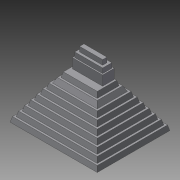
# Autodesk Inventor part: Basic Temple
Saved by Autodesk Inventor 2015 (Build 190159000, 159)
## iProperties
Created: 2016-11-16
Part Number: Basic Temple
Material: Generic
Document SubType Name: Modeling
Designer: Simms
Density: 1 g/cm^3
Appearance: Default
Author: Simms
Autodesk Inventor part; units mm, degrees
ref_plane "YZ Plane" through (0, 0, 0) normal (1, 0, 0) x (0, 1, 0)
ref_plane "XY Plane" through (0, 0, 0) normal (0, 0, 1) x (1, 0, 0)
sketch "Sketch1" plane through (0, 0, 0) normal (0, 1, 0) x (-1, 0, 0)
  line L0 (-228.6, 190.5) -> (228.6, 190.5)
  line L1 (228.6, 190.5) -> (228.6, -190.5)
  line L2 (228.6, -190.5) -> (-228.6, -190.5)
  line L3 (-228.6, -190.5) -> (-228.6, 190.5)
  line L4 (-228.6, 190.5) -> (228.6, -190.5) construction
  line L5 (228.6, 190.5) -> (-228.6, -190.5) construction
  point P0 (0, 0)
  dimension "d0" = 457.2
  dimension "d1" = 381
  constraints: 12 end point, 2 midpoint, 2 parallel, 1 horizontal, 1 perpendicular
  measures "d0" distance of L1.end L2.end
  measures "d1" distance of L0.end L1.end
ref_plane "Work Plane1" through (0, 25.4, 0) normal (0, 1, 0) x (-1, 0, 0)
pattern_of_nothing "Rectangular Pattern1"
sketch "Sketch2" plane through (0, 25.4, 0) normal (0, 1, 0) x (-1, 0, 0)
  line L0 (228.6, 190.5) -> (228.6, -190.5) projected
  line L1 (228.6, -190.5) -> (-228.6, -190.5) projected
  line L2 (-228.6, -190.5) -> (-228.6, 190.5) projected
  line L3 (-228.6, 190.5) -> (228.6, 190.5) projected
  line L4 (222.25, -184.15) -> (222.25, 184.15)
  line L5 (222.25, 184.15) -> (-222.25, 184.15)
  line L6 (-222.25, 184.15) -> (-222.25, -184.15)
  line L7 (-222.25, -184.15) -> (222.25, -184.15)
  point P0 (0, 0)
  dimension "d7" = 6.35
  constraints: 8 end point, 3 other
  measures "d7" distance between parallel lines of L0 L4
loft "Loft1" add profiles "Sketch1", "Sketch2" contours all / L7 L6 L5 L4
sketch "Sketch4" plane through (0, 25.4, 0) normal (0, 1, 0) x (-1, 0, 0)
  line L0 (222.25, 184.15) -> (222.25, -184.15) projected
  line L1 (-222.25, 184.15) -> (222.25, 184.15) projected
  line L2 (-222.25, -184.15) -> (-222.25, 184.15) projected
  line L3 (222.25, -184.15) -> (-222.25, -184.15) projected
  line L4 (222.25, 184.15) -> (222.25, -184.15) projected
  line L5 (-212.725, -174.625) -> (-212.725, 174.625)
  line L6 (-212.725, 174.625) -> (212.725, 174.625)
  line L7 (212.725, 174.625) -> (212.725, -174.625)
  line L8 (212.725, -174.625) -> (-212.725, -174.625)
  point P0 (0, 0)
  dimension "d12" = 9.525
  constraints: 8 end point, 3 other
  measures "d12" distance between parallel lines of L3 L8
sketch "Sketch5" plane through (0, 50.8, 0) normal (0, 1, 0) x (-1, 0, 0)
  line L0 (212.725, 174.625) -> (212.725, -174.625) projected
  line L1 (212.725, -174.625) -> (-212.725, -174.625) projected
  line L2 (-212.725, -174.625) -> (-212.725, 174.625) projected
  line L3 (-212.725, 174.625) -> (212.725, 174.625) projected
  line L4 (-206.375, -168.275) -> (206.375, -168.275)
  line L5 (206.375, -168.275) -> (206.375, 168.275)
  line L6 (206.375, 168.275) -> (-206.375, 168.275)
  line L7 (-206.375, 168.275) -> (-206.375, -168.275)
  point P0 (0, 0)
  dimension "d13" = 6.35
  constraints: 8 end point, 3 other
  measures "d13" distance between parallel lines of L1 L4
sketch "Sketch6" plane through (0, 50.8, 0) normal (0, 1, 0) x (-1, 0, 0)
  line L0 (-206.375, -168.275) -> (206.375, -168.275) projected
  line L1 (206.375, -168.275) -> (206.375, 168.275) projected
  line L2 (-206.375, 168.275) -> (-206.375, -168.275) projected
  line L3 (206.375, 168.275) -> (-206.375, 168.275) projected
  line L4 (196.85, -158.75) -> (-196.85, -158.75)
  line L5 (-196.85, -158.75) -> (-196.85, 158.75)
  line L6 (-196.85, 158.75) -> (196.85, 158.75)
  line L7 (196.85, 158.75) -> (196.85, -158.75)
  point P0 (0, 0)
  dimension "d14" = 9.525
  constraints: 8 end point, 3 other
  measures "d14" distance between parallel lines of L0 L4
loft "Loft2" add profiles "Sketch4", "Sketch5" contours L5 L6 L7 L8 / L7 L6 L5 L4
sketch "Sketch7" plane through (0, 76.2, 0) normal (0, 1, 0) x (-1, 0, 0)
  line L0 (196.85, -158.75) -> (-196.85, -158.75) projected
  line L1 (196.85, 158.75) -> (196.85, -158.75) projected
  line L2 (-196.85, 158.75) -> (196.85, 158.75) projected
  line L3 (-196.85, -158.75) -> (-196.85, 158.75) projected
  line L4 (-190.5, -152.4) -> (190.5, -152.4)
  line L5 (190.5, -152.4) -> (190.5, 152.4)
  line L6 (190.5, 152.4) -> (-190.5, 152.4)
  line L7 (-190.5, 152.4) -> (-190.5, -152.4)
  point P0 (0, 0)
  dimension "d19" = 6.35
  constraints: 8 end point, 3 other
  measures "d19" distance between parallel lines of L0 L4
loft "Loft3" add profiles "Sketch6", "Sketch7" contours L4 L5 L6 L7 / L7 L6 L5 L4
sketch "Sketch8" plane through (0, 76.2, 0) normal (0, 1, 0) x (-1, 0, 0)
  line L0 (190.5, -152.4) -> (-190.5, -152.4) projected
  line L1 (190.5, 152.4) -> (190.5, -152.4) projected
  line L2 (-190.5, 152.4) -> (190.5, 152.4) projected
  line L3 (-190.5, -152.4) -> (-190.5, 152.4) projected
  line L4 (-180.975, -142.875) -> (180.975, -142.875)
  line L5 (180.975, -142.875) -> (180.975, 142.875)
  line L6 (180.975, 142.875) -> (-180.975, 142.875)
  line L7 (-180.975, 142.875) -> (-180.975, -142.875)
  point P0 (0, 0)
  dimension "d24" = 9.525
  constraints: 8 end point, 3 other
  measures "d24" distance between parallel lines of L0 L4
sketch "Sketch9" plane through (0, 101.6, 0) normal (0, 1, 0) x (-1, 0, 0)
  line L0 (-180.975, -142.875) -> (180.975, -142.875) projected
  line L1 (180.975, -142.875) -> (180.975, 142.875) projected
  line L2 (180.975, 142.875) -> (-180.975, 142.875) projected
  line L3 (-180.975, 142.875) -> (-180.975, -142.875) projected
  line L4 (174.625, -136.525) -> (-174.625, -136.525)
  line L5 (-174.625, -136.525) -> (-174.625, 136.525)
  line L6 (-174.625, 136.525) -> (174.625, 136.525)
  line L7 (174.625, 136.525) -> (174.625, -136.525)
  point P0 (0, 0)
  dimension "d25" = 6.35
  constraints: 8 end point, 3 other
  measures "d25" distance between parallel lines of L0 L4
loft "Loft4" add profiles "Sketch8", "Sketch9" contours L7 L6 L5 L4 / L4 L5 L6 L7
sketch "Sketch10" plane through (0, 101.6, 0) normal (0, 1, 0) x (-1, 0, 0)
  line L0 (-174.625, -136.525) -> (174.625, -136.525) projected
  line L1 (174.625, -136.525) -> (174.625, 136.525) projected
  line L2 (174.625, 136.525) -> (-174.625, 136.525) projected
  line L3 (-174.625, 136.525) -> (-174.625, -136.525) projected
  line L4 (165.1, -127) -> (-165.1, -127)
  line L5 (-165.1, -127) -> (-165.1, 127)
  line L6 (-165.1, 127) -> (165.1, 127)
  line L7 (165.1, 127) -> (165.1, -127)
  point P0 (0, 0)
  dimension "d30" = 9.525
  constraints: 8 end point, 3 other
  measures "d30" distance between parallel lines of L0 L4
sketch "Sketch11" plane through (0, 127, 0) normal (0, 1, 0) x (-1, 0, 0)
  line L0 (165.1, -127) -> (-165.1, -127) projected
  line L1 (165.1, 127) -> (165.1, -127) projected
  line L2 (-165.1, 127) -> (165.1, 127) projected
  line L3 (-165.1, -127) -> (-165.1, 127) projected
  line L4 (-158.75, -120.65) -> (158.75, -120.65)
  line L5 (158.75, -120.65) -> (158.75, 120.65)
  line L6 (158.75, 120.65) -> (-158.75, 120.65)
  line L7 (-158.75, 120.65) -> (-158.75, -120.65)
  point P0 (0, 0)
  dimension "d31" = 6.35
  constraints: 8 end point, 3 other
  measures "d31" distance between parallel lines of L0 L4
loft "Loft5" add profiles "Sketch10", "Sketch11" contours L4 L5 L6 L7 / L7 L6 L5 L4
sketch "Sketch13" plane through (0, 127, 0) normal (0, 1, 0) x (-1, 0, 0)
  line L0 (158.75, -120.65) -> (-158.75, -120.65) projected
  line L1 (158.75, 120.65) -> (158.75, -120.65) projected
  line L2 (-158.75, 120.65) -> (158.75, 120.65) projected
  line L3 (-158.75, -120.65) -> (-158.75, 120.65) projected
  line L4 (-149.225, -111.125) -> (149.225, -111.125)
  line L5 (149.225, -111.125) -> (149.225, 111.125)
  line L6 (149.225, 111.125) -> (-149.225, 111.125)
  line L7 (-149.225, 111.125) -> (-149.225, -111.125)
  point P0 (0, 0)
  dimension "d36" = 9.525
  constraints: 8 end point, 3 other
  measures "d36" distance between parallel lines of L0 L4
sketch "Sketch14" plane through (0, 152.4, 0) normal (0, 1, 0) x (-1, 0, 0)
  line L0 (149.225, -111.125) -> (149.225, 111.125) projected
  line L1 (-149.225, -111.125) -> (149.225, -111.125) projected
  line L2 (149.225, 111.125) -> (-149.225, 111.125) projected
  line L3 (-149.225, 111.125) -> (-149.225, -111.125) projected
  line L4 (142.875, -104.775) -> (142.875, 104.775)
  line L5 (142.875, 104.775) -> (-142.875, 104.775)
  line L6 (-142.875, 104.775) -> (-142.875, -104.775)
  line L7 (-142.875, -104.775) -> (142.875, -104.775)
  point P0 (0, 0)
  dimension "d37" = 6.35
  constraints: 8 end point, 3 other
  measures "d37" distance between parallel lines of L1 L7
loft "Loft6" add profiles "Sketch13", "Sketch14" contours L7 L6 L5 L4 / L7 L6 L5 L4
sketch "Sketch15" plane through (0, 152.4, 0) normal (0, 1, 0) x (-1, 0, 0)
  line L0 (-142.875, -104.775) -> (142.875, -104.775) projected
  line L1 (142.875, -104.775) -> (142.875, 104.775) projected
  line L2 (142.875, 104.775) -> (-142.875, 104.775) projected
  line L3 (-142.875, 104.775) -> (-142.875, -104.775) projected
  line L4 (133.35, -95.25) -> (-133.35, -95.25)
  line L5 (-133.35, -95.25) -> (-133.35, 95.25)
  line L6 (-133.35, 95.25) -> (133.35, 95.25)
  line L7 (133.35, 95.25) -> (133.35, -95.25)
  point P0 (0, 0)
  dimension "d42" = 9.525
  constraints: 8 end point, 3 other
  measures "d42" distance between parallel lines of L0 L4
sketch "Sketch16" plane through (0, 177.8, 0) normal (0, 1, 0) x (-1, 0, 0)
  line L0 (133.35, 95.25) -> (133.35, -95.25) projected
  line L1 (133.35, -95.25) -> (-133.35, -95.25) projected
  line L2 (-133.35, 95.25) -> (133.35, 95.25) projected
  line L3 (-133.35, -95.25) -> (-133.35, 95.25) projected
  line L4 (-127, -88.9) -> (127, -88.9)
  line L5 (127, -88.9) -> (127, 88.9)
  line L6 (127, 88.9) -> (-127, 88.9)
  line L7 (-127, 88.9) -> (-127, -88.9)
  point P0 (0, 0)
  dimension "d43" = 6.35
  constraints: 8 end point, 3 other
  measures "d43" distance between parallel lines of L1 L4
loft "Loft7" add profiles "Sketch15", "Sketch16" contours L4 L5 L6 L7 / L7 L6 L5 L4
sketch "Sketch17" plane through (0, 177.8, 0) normal (0, 1, 0) x (-1, 0, 0)
  line L0 (127, -88.9) -> (-127, -88.9) projected
  line L1 (127, 88.9) -> (127, -88.9) projected
  line L2 (-127, 88.9) -> (127, 88.9) projected
  line L3 (-127, -88.9) -> (-127, 88.9) projected
  line L4 (-117.475, -79.375) -> (117.475, -79.375)
  line L5 (117.475, -79.375) -> (117.475, 79.375)
  line L6 (117.475, 79.375) -> (-117.475, 79.375)
  line L7 (-117.475, 79.375) -> (-117.475, -79.375)
  point P0 (0, 0)
  dimension "d48" = 9.525
  constraints: 8 end point, 3 other
  measures "d48" distance between parallel lines of L0 L4
sketch "Sketch18" plane through (0, 203.2, 0) normal (0, 1, 0) x (-1, 0, 0)
  line L0 (117.475, -79.375) -> (117.475, 79.375) projected
  line L1 (-117.475, -79.375) -> (117.475, -79.375) projected
  line L2 (117.475, 79.375) -> (-117.475, 79.375) projected
  line L3 (-117.475, 79.375) -> (-117.475, -79.375) projected
  line L4 (104.775, -66.675) -> (104.775, 66.675)
  line L5 (104.775, 66.675) -> (-104.775, 66.675)
  line L6 (-104.775, 66.675) -> (-104.775, -66.675)
  line L7 (-104.775, -66.675) -> (104.775, -66.675)
  point P0 (0, 0)
  dimension "d49" = 12.7
  constraints: 8 end point, 3 other
  measures "d49" distance between parallel lines of L1 L7
loft "Loft8" add profiles "Sketch17", "Sketch18" contours L7 L6 L5 L4 / L7 L6 L5 L4
sketch "Sketch19" plane through (0, 203.2, 0) normal (0, 1, 0) x (-1, 0, 0)
  line L0 (-104.775, -66.675) -> (104.775, -66.675) projected
  line L1 (104.775, -66.675) -> (104.775, 66.675) projected
  line L2 (104.775, 66.675) -> (-104.775, 66.675) projected
  line L3 (-104.775, 66.675) -> (-104.775, -66.675) projected
  line L4 (95.25, -57.15) -> (-95.25, -57.15)
  line L5 (-95.25, -57.15) -> (-95.25, 57.15)
  line L6 (-95.25, 57.15) -> (95.25, 57.15)
  line L7 (95.25, 57.15) -> (95.25, -57.15)
  point P0 (0, 0)
  dimension "d54" = 9.525
  constraints: 8 end point, 3 other
  measures "d54" distance between parallel lines of L0 L4
sketch "Sketch20" plane through (0, 228.6, 0) normal (0, 1, 0) x (-1, 0, 0)
  line L0 (95.25, 57.15) -> (95.25, -57.15) projected
  line L1 (95.25, -57.15) -> (-95.25, -57.15) projected
  line L2 (-95.25, 57.15) -> (95.25, 57.15) projected
  line L3 (-95.25, -57.15) -> (-95.25, 57.15) projected
  line L4 (-88.9, -50.8) -> (88.9, -50.8)
  line L5 (88.9, -50.8) -> (88.9, 50.8)
  line L6 (88.9, 50.8) -> (-88.9, 50.8)
  line L7 (-88.9, 50.8) -> (-88.9, -50.8)
  point P0 (0, 0)
  dimension "d55" = 6.35
  constraints: 8 end point, 3 other
  measures "d55" distance between parallel lines of L1 L4
loft "Loft9" add profiles "Sketch19", "Sketch20" contours L4 L5 L6 L7 / L7 L6 L5 L4
sketch "Sketch21" plane through (-88.9, 228.6, -50.8) normal (0, 1, 0) x (1, 0, 0)
  line L0 (9.525, -3.175) -> (168.275, -3.175)
  line L1 (168.275, -3.175) -> (168.275, -63.9699)
  line L2 (168.275, -63.9699) -> (9.525, -63.9699)
  line L3 (9.525, -63.9699) -> (9.525, -3.175)
  line L4 (177.8, 0) -> (177.8, -101.6) projected
  line L5 (0, -101.6) -> (0, 0) projected
  line L6 (0, 0) -> (177.8, 0) projected
  point P0 (88.9, -50.8)
  dimension "d60" = 9.525
  dimension "d61" = 9.525
  dimension "d62" = 3.175
  constraints: 8 end point, 2 parallel, 1 horizontal, 1 perpendicular
  measures "d60" distance between parallel lines of L4 L1
  measures "d61" distance between parallel lines of L5 L3
  measures "d62" distance between parallel lines of L0 L6
extrude "Extrusion1" add sketch "Sketch21" along normal blind 50.8
sketch "Sketch22" plane through (-88.9, 279.4, -50.8) normal (0, 1, 0) x (1, 0, 0)
  line L0 (168.275, -3.175) -> (9.525, -3.175) projected
  line L1 (9.525, -3.175) -> (9.525, -63.9699) projected
  line L2 (9.525, -63.9699) -> (168.275, -63.9699) projected
  line L3 (168.275, -63.9699) -> (168.275, -3.175) projected
  line L4 (15.875, -9.525) -> (161.925, -9.525)
  line L5 (161.925, -9.525) -> (161.925, -57.6199)
  line L6 (161.925, -57.6199) -> (15.875, -57.6199)
  line L7 (15.875, -57.6199) -> (15.875, -9.525)
  point P0 (88.9, -50.8)
  dimension "d65" = 6.35
  constraints: 8 end point, 3 other
  measures "d65" distance between parallel lines of L0 L4
extrude "Extrusion2" add sketch "Sketch22" along normal blind 25.4 contours L4 L5 L6 L7
sketch "Sketch23" plane through (-88.9, 304.8, -50.8) normal (0, 1, 0) x (1, 0, 0)
  line L0 (161.925, -9.525) -> (15.875, -9.525) projected
  line L1 (15.875, -9.525) -> (15.875, -57.6199) projected
  line L2 (15.875, -57.6199) -> (161.925, -57.6199) projected
  line L3 (161.925, -57.6199) -> (161.925, -9.525) projected
  line L4 (28.575, -22.225) -> (149.225, -22.225)
  line L5 (149.225, -22.225) -> (149.225, -44.9199)
  line L6 (149.225, -44.9199) -> (28.575, -44.9199)
  line L7 (28.575, -44.9199) -> (28.575, -22.225)
  point P0 (88.9, -50.8)
  dimension "d68" = 12.7
  constraints: 8 end point, 3 other
  measures "d68" distance between parallel lines of L0 L4
extrude "Extrusion3" add sketch "Sketch23" along normal blind 25.4 contours L4 L5 L6 L7
ref_plane "Work Plane3" through (0, 50.8, 0) normal (0, 1, 0) x (-1, 0, 0)
ref_plane "Work Plane4" through (0, 76.2, 0) normal (0, 1, 0) x (-1, 0, 0)
ref_plane "Work Plane5" through (0, 101.6, 0) normal (0, 1, 0) x (-1, 0, 0)
ref_plane "Work Plane6" through (0, 127, 0) normal (0, 1, 0) x (-1, 0, 0)
ref_plane "Work Plane7" through (0, 152.4, 0) normal (0, 1, 0) x (-1, 0, 0)
ref_plane "Work Plane8" through (0, 177.8, 0) normal (0, 1, 0) x (-1, 0, 0)
ref_plane "Work Plane9" through (0, 203.2, 0) normal (0, 1, 0) x (-1, 0, 0)
ref_plane "Work Plane10" through (0, 228.6, 0) normal (0, 1, 0) x (-1, 0, 0)
body "Solid1"
